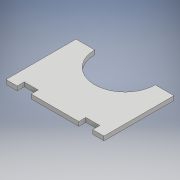
# Autodesk Inventor part: Support_motor_front_2
Saved by Autodesk Inventor 2017 (Build 210142000, 142)
## iProperties
Part Number: Support_motor_front_2
Material: Générique
Document SubType Name: Modeling
Designer: Darren
Density: 1 g/cm^3
Appearance: Par défaut
Author: Darren
Autodesk Inventor part; units mm, degrees
ref_plane "YZ Plane" through (0, 0, 0) normal (1, 0, 0) x (0, 1, 0)
ref_plane "XZ Plane" through (0, 0, 0) normal (0, 1, 0) x (-1, 0, 0)
ref_plane "XY Plane" through (0, 0, 0) normal (0, 0, 1) x (1, 0, 0)
sketch "Esquisse1" plane through (0, 0, 0) normal (0, 0, 1) x (1, 0, 0)
  line L0 (0, -14) -> (0, 14) construction
  circle A0 centre (0, 0) radius 30 construction
  line L1 (0, 0) -> (35, 0) construction
  line L2 (0, 0) -> (-35, 0) construction
  line L3 (-35, 0) -> (35, 0) construction
  line L4 (35, 0) -> (35, -50)
  line L5 (-35, -50) -> (-35, 0)
  line L6 (-49, 0) -> (49, 0) construction
  line L7 (0, -66) -> (0, 46) construction
  arc A1 (-21.6, 0) -> (21.6, 0) centre (0, 0) ccw
  line L8 (-35, 0) -> (-21.6, 0)
  line L9 (35, 0) -> (21.6, 0)
  line L10 (-17, -50) -> (-17, -45)
  line L11 (-17, -45) -> (-27, -45)
  line L12 (-27, -45) -> (-27, -50)
  line L13 (27, -50) -> (27, -45)
  line L14 (27, -45) -> (17, -45)
  line L15 (17, -45) -> (17, -50)
  line L16 (-27, -50) -> (-35, -50)
  line L17 (35, -50) -> (27, -50)
  line L18 (17, -50) -> (-17, -50)
  line L19 (0, 0) -> (21.6, 0) construction
  line L20 (30, 0) -> (35, 0) construction
  dimension "d8" = 60
  dimension "d12" = 70
  dimension "d23" = 35
  dimension "d25" = 21.6
  dimension "d26" = 10
  dimension "d28" = 10
  dimension "d30" = 8
  dimension "d31" = 8
  dimension "d32" = 5
  dimension "d33" = 5
  dimension "d34" = 5
  dimension "d35" = 50
  dimension "d36" = 5
  constraints: 38 end point, 7 parallel, 2 coincident, 2 horizontal, 2 midpoint, 2 point on circle, 2 point on line, 1 centre point, 1 collinear, 1 horizontal alignment, 1 perpendicular, 2 other
  measures "d12" distance of L4.end L5.start
  measures "d23" distance between parallel lines of L7 L5
  measures "d25" radius of A1
  measures "d26" distance of L11.end L10.end
  measures "d28" distance of L14.end L13.end
  measures "d30" distance between parallel lines of L4 L13
  measures "d31" distance between parallel lines of L5 L12
  measures "d32" distance between parallel lines of L18 L11
  measures "d33" distance between parallel lines of L18 L14
  measures "d34" distance between parallel lines of L17 L14
  measures "d35" distance between parallel lines of L17 L6
  measures "d36" distance between parallel lines of L11 L16
extrude "Extrusion1" add sketch "Esquisse1" along normal blind 3
